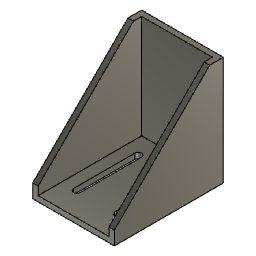
Equerre (Autodesk Fusion 360 design; units mm, degrees)
Autodesk Fusion 360 part; units mm, degrees
sketch "Sketch2" plane through (0, 0, 0) normal (0, 0, 1) x (1, 0, 0)
  line L0 (0, 0) -> (60, 0)
  line L1 (60, 0) -> (60, 80)
  line L2 (60, 80) -> (0, 80)
  line L3 (0, 80) -> (0, 0)
  line L4 (56, 0) -> (56, 76)
  line L5 (56, 76) -> (4, 76)
  line L6 (4, 76) -> (4, 0)
  line L7 (15, 65) -> (15, 65)
  line L8 (17.5, 62.5) -> (17.5, 17.5)
  line L9 (15, 15) -> (15, 15)
  line L10 (12.5, 17.5) -> (12.5, 62.5)
  line L11 (45, 65) -> (45, 65)
  line L12 (47.5, 62.5) -> (47.5, 17.5)
  line L13 (45, 15) -> (45, 15)
  line L14 (42.5, 17.5) -> (42.5, 62.5)
  arc A0 (15, 65) -> (12.5, 62.5) centre (15, 62.5) ccw
  arc A1 (17.5, 62.5) -> (15, 65) centre (15, 62.5) ccw
  arc A2 (45, 65) -> (42.5, 62.5) centre (45, 62.5) ccw
  arc A3 (47.5, 62.5) -> (45, 65) centre (45, 62.5) ccw
  arc A4 (12.5, 17.5) -> (15, 15) centre (15, 17.5) ccw
  arc A5 (15, 15) -> (17.5, 17.5) centre (15, 17.5) ccw
  arc A6 (42.5, 17.5) -> (45, 15) centre (45, 17.5) ccw
  arc A7 (45, 15) -> (47.5, 17.5) centre (45, 17.5) ccw
  dimension "d1" = 60
  dimension "d2" = 80
  dimension "d3" = 4
  dimension "d4" = 4
  dimension "d5" = 4
  dimension "d7" = 25
  dimension "d8" = 8.5
  dimension "d9" = 5
  dimension "d10" = 5
  dimension "d14" = 2.5
  dimension "d15" = 2.5
  dimension "d16" = 2.5
  dimension "d17" = 2.5
  dimension "d18" = 2.5
  dimension "d19" = 2.5
  dimension "d20" = 15
  constraint horizontal L0
  constraint vertical L1
  constraint horizontal L2
  constraint vertical L3
  constraint coincident L0.start L3.end
  constraint vertical L4
  constraint horizontal L5
  constraint vertical L6
  constraint coincident L0 L6.end
  constraint vertical L8
  constraint vertical L10
  constraint vertical L12
  constraint vertical L14
  constraint tangent L10 A0
  constraint tangent L8 A1
  constraint tangent L14 A2
  constraint tangent L12 A3
  constraint tangent L10 A4
  constraint tangent L8 A5
  constraint equal A4 A5
  constraint tangent L14 A6
  constraint tangent L12 A7
  constraint equal A6 A7
  measures "d1" distance of L1 L3
  measures "d2" distance of L0 L2
  measures "d3" distance of L2 L5
  measures "d4" distance of L1 L4
  measures "d5" distance of L3 L6
  measures "d7" distance of L8 L14
  measures "d8" distance of L6 L10
  measures "d9" distance of L8 L10
  measures "d10" distance of L12 L14
  measures "d14" radius of A0
  measures "d15" radius of A1
  measures "d17" radius of A3
  measures "d18" radius of A4
  measures "d19" radius of A6
  measures "d20" distance of L0 L9.start
extrude "Extrude1" add sketch "Sketch2" along normal blind 4 contours L0 L1 L2 L3 L4 L5 L6 | L0 L4 L5 L6 | L8 L10 A0 A1 A4 A5 | L12 L14 A2 A3 A6 A7
extrude "Extrude2" add sketch "Sketch2" along normal blind 80 contours L0 L1 L2 L3 L4 L5 L6
sketch "Sketch3" plane through (60, 0, 0) normal (1, 0, 0) x (0, 1, 0)
  line L0 (0, 0) -> (80, 0)
  line L1 (80, 0) -> (80, 80)
  line L2 (80, 80) -> (0, 80)
  line L3 (0, 80) -> (0, 0)
  line L4 (0, 10) -> (70, 80)
  dimension "d25" = 10
  dimension "d26" = 10
  constraint coincident L3 L4.start
  constraint coincident L2 L4.end
  measures "d25" distance of L1 L4.end
  measures "d26" distance of L0 L4.start
extrude "Extrude3" cut sketch "Sketch3" against normal blind 95 contours L2 L3 L4
extrude "Extrude4" cut sketch "Sketch2" along normal blind 10 contours L8 L10 A0 A1 A4 A5 | L12 L14 A2 A3 A6 A7
